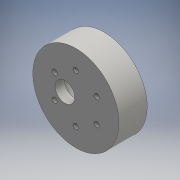
# Autodesk Inventor part: motor_holder_test
Saved by Autodesk Inventor 2016 (Build 200138000, 138)
## iProperties
Created: 2017-03-03
Part Number: motor_holder_test
Material: Generic
Document SubType Name: Modeling
Designer: Samuelsson
Density: 1 g/cm^3
Appearance: Default
Author: Samuelsson
Autodesk Inventor part; units mm, degrees
ref_plane "YZ Plane" through (0, 0, 0) normal (1, 0, 0) x (0, 1, 0)
ref_plane "XZ Plane" through (0, 0, 0) normal (0, 1, 0) x (-1, 0, 0)
ref_plane "XY Plane" through (0, 0, 0) normal (0, 0, 1) x (1, 0, 0)
sketch "Sketch1" plane through (0, 0, 0) normal (0, 1, 0) x (-1, 0, 0)
  circle A0 centre (7, 0) radius 6.25
  circle A1 centre (0, 15.5) radius 1.6
  circle A2 centre (-13.4234, 7.75) radius 1.6
  circle A3 centre (-13.4234, -7.75) radius 1.6
  circle A4 centre (0, -15.5) radius 1.6
  circle A5 centre (13.4234, -7.75) radius 1.6
  circle A6 centre (13.4234, 7.75) radius 1.6
  circle A7 centre (0, 0) radius 27.5
  dimension "d0" = 7
  dimension "d1" = 12.5
  dimension "d2" = 3.2
  dimension "d3" = 15.5
  dimension "d6" = 360
  dimension "d8" = 55
  constraints: 8 centre point, 1 coincident, 1 horizontal alignment, 1 vertical alignment, 13 other
  measures "d0" distance of point (0, 0) A0.centre
  measures "d1" diameter of A0
  measures "d2" diameter of A1
  measures "d3" distance of point (0, 0) A1.centre
  measures "d8" diameter of A7
extrude "Extrusion1" add sketch "Sketch1" along normal blind 6
sketch "Sketch2" plane through (0, 6, 0) normal (0, 1, 0) x (1, 0, 0)
  circle A0 centre (0, 0) radius 19
  circle A1 centre (0, 0) radius 27.5
  dimension "d11" = 38
  constraints: 2 centre point, 2 coincident
  measures "d11" diameter of A0
extrude "Extrusion2" add sketch "Sketch2" along normal blind 12
body "Solid1"
